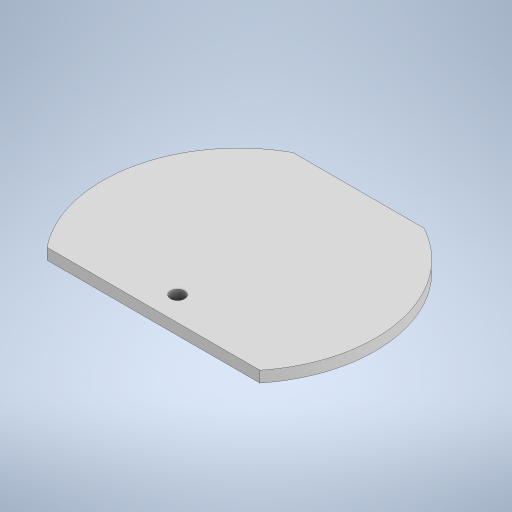
# Autodesk Inventor part: huta
Saved by Autodesk Inventor 2024 (Build 280153000, 153)
## iProperties
Created: 2024-02-22
Part Number: huta
Material: 一般
Document SubType Name: Modeling
Designer: mott1
Density: 1 g/cm^3
Appearance: 既定
Author: mott1
Autodesk Inventor part; units mm, degrees
ref_plane "YZ Plane" through (0, 0, 0) normal (1, 0, 0) x (0, 1, 0)
ref_plane "XZ Plane" through (0, 0, 0) normal (0, 1, 0) x (-1, 0, 0)
ref_plane "XY Plane" through (0, 0, 0) normal (0, 0, 1) x (1, 0, 0)
sketch "スケッチ1" plane through (0, 0, 0) normal (0, 1, 0) x (-1, 0, 0)
  point P0 (0, 0)
sketch "スケッチ2" plane through (0, 0, 0) normal (0, 1, 0) x (-1, 0, 0)
  arc A0 (-19.1073, 15.335) -> (-11.7473, -21.5) centre (0, 0) ccw
  line L0 (0, 0) -> (0, -21.5)
  line L1 (0, 0) -> (0, 15.335)
  line L2 (0, -21.5) -> (-11.7473, -21.5)
  line L3 (0, 15.335) -> (-19.1073, 15.335)
  dimension "d1" = 21.5
  dimension "d3" = 15.335
  dimension "d4" = 24.5
  constraints: 8 end point, 2 point on circle, 2 vertical, 1 centre point, 1 coincident, 1 horizontal, 1 parallel
  measures "d1" distance of L0.start L0.end
  measures "d3" distance of L0.start L1.end
  measures "d4" radius of A0
extrude "押し出し1" add sketch "スケッチ2" along normal blind 2
sketch "スケッチ3" plane through (0, 2, 0) normal (0, 1, 0) x (1, 0, 0)
  line L0 (0, 21.5) -> (0, -15.335) projected
  circle A0 centre (0, -11) radius 1.25
  point P0 (0, 0)
  point P1 (0, -9.75)
  point P2 (0, -12.25)
  dimension "d7" = 2.5
  dimension "d8" = 11
  constraints: 1 centre point, 1 point on line
  measures "d7" diameter of A0
  measures "d8" distance of A0.centre point (0, 0)
extrude "押し出し2" cut sketch "スケッチ3" against normal blind 10 contours A0 L0 picked at (0.1808, -10.6246)
mirror "ミラー2" about plane through (0, 0, -21.5) normal (-1, 0, 0) of "押し出し2", "押し出し1"
